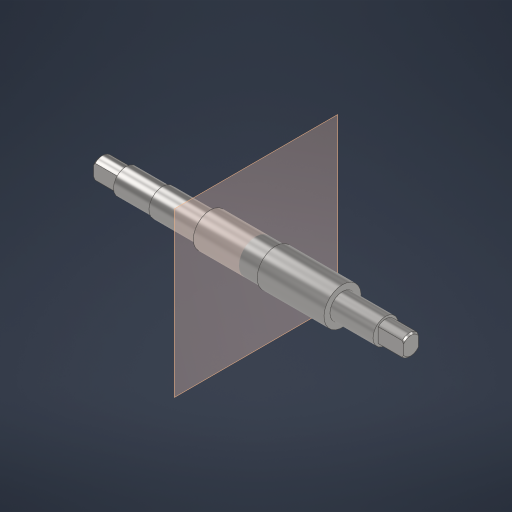
# Autodesk Inventor part: axel
Saved by Autodesk Inventor 2024 (Build 280153000, 153)
## iProperties
Created: 2024-04-30
Part Number: axel
Material: Stainless Steel
Document SubType Name: Modeling
Designer: markm
Density: 8 g/cm^3
Appearance: Semi-Polished
Author: markm
Autodesk Inventor part; units mm, degrees
ref_plane "YZ Plane" through (0, 0, 0) normal (1, 0, 0) x (0, 1, 0)
ref_plane "XZ Plane" through (0, 0, 0) normal (0, 1, 0) x (-1, 0, 0)
ref_plane "XY Plane" through (0, 0, 0) normal (0, 0, 1) x (1, 0, 0)
sketch "Sketch4" plane through (0, 0, 0) normal (0, 0, 1) x (1, 0, 0)
  line L0 (-102.025, 0) -> (106.725, 0)
  line L1 (-28.375, 11.5) -> (15.625, 11.5)
  line L2 (15.625, 11.5) -> (15.625, 12.5)
  line L3 (15.625, 12.5) -> (60.625, 12.5)
  line L4 (60.625, 12.5) -> (60.625, 8.5)
  line L5 (60.625, 8.5) -> (89.625, 8.5)
  line L6 (89.625, 8.5) -> (89.625, 7)
  line L7 (89.625, 7) -> (106.725, 7)
  line L8 (106.725, 7) -> (106.725, 0)
  line L9 (-28.375, 11.5) -> (-28.375, 9.125)
  line L10 (-28.375, 9.125) -> (-60.625, 9.125)
  line L11 (-60.625, 9.125) -> (-60.625, 8.5)
  line L12 (-60.625, 8.5) -> (-85.125, 8.5)
  line L13 (-85.125, 8.5) -> (-85.125, 7)
  line L14 (-85.125, 7) -> (-102.025, 7)
  line L15 (-102.025, 7) -> (-102.025, 0)
  line L16 (0, 0) -> (0, 42.8251) construction
  dimension "d12" = 14
  dimension "d13" = 17
  dimension "d16" = 23
  dimension "d18" = 25
  dimension "d20" = 18.25
  dimension "d30" = 89
  dimension "d31" = 45
  dimension "d32" = 29
  dimension "d33" = 17.1
  dimension "d34" = 32.25
  dimension "d35" = 24.5
  dimension "d36" = 16.9
  constraints: 34 end point, 13 perpendicular, 2 collinear, 2 horizontal, 2 vertical, 1 point on line, 1 other
  measures "d12" diameter of L7 L0
  measures "d13" diameter of L5 L0
  measures "d16" diameter of L1 L0
  measures "d18" diameter of L3 L0
  measures "d20" diameter of L10 L0
  measures "d30" distance between parallel lines of L4 L9
  measures "d31" distance of L2.end L3.end
  measures "d32" distance of L4.end L5.end
  measures "d33" distance of L6.end L7.end
  measures "d34" distance of L9.end L10.end
  measures "d35" distance of L11.end L12.end
  measures "d36" distance of L13.end L14.end
revolve "Revolution1" add sketch "Sketch4" angle 360 about axis through (-102.025, 0, 0) along (1, 0, 0)
chamfer "Chamfer1" distance 1 angle 45 2 edges at (106.725, -7, 0) (-102.025, -7, 0)
sketch "Sketch5" plane through (106.725, 0, 0) normal (1, 0, 0) x (0, 0, -1)
  circle A0 centre (0, 0) radius 7 projected
  line L0 (-5, 4.899) -> (-5, -4.899)
  line L1 (5, -4.899) -> (5, 4.899)
  point P0 (0, 0)
  dimension "d27" = 10
  constraints: 4 end point, 4 point on circle, 2 parallel, 1 vertical
  measures "d27" distance between parallel lines of L1 L0
extrude "Extrusion4" cut sketch "Sketch5" against normal up to surface (17.1 mm away) contours A0 L1 | L0 A0
ref_plane "Work Plane1" through (2.35, -3.3166, -5) normal (1, 0, 0) x (0, 0, -1)
mirror "Mirror1" about plane through (2.35, -3.3166, -5) normal (1, 0, 0) of "Extrusion4"
body "Solid2"
